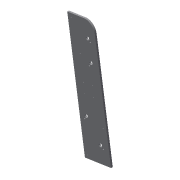
# Autodesk Inventor part: inside wall
Saved by Autodesk Inventor 2020 (Build 240168000, 168)
## iProperties
Created: 2019-10-13
Part Number: inside wall
Material: Generic
Document SubType Name: Modeling
Designer: ball
Density: 1 g/cm^3
Appearance: Default
Author: ball
Autodesk Inventor part; units mm, degrees
ref_plane "YZ Plane" through (0, 0, 0) normal (1, 0, 0) x (0, 1, 0)
ref_plane "XZ Plane" through (0, 0, 0) normal (0, 1, 0) x (-1, 0, 0)
ref_plane "XY Plane" through (0, 0, 0) normal (0, 0, 1) x (1, 0, 0)
ref_plane "Work Plane1" through (-0.0003, 0.0023, 0) normal (0, 0, 1) x (1, 0, 0)
sketch "Sketch1" plane through (-0.0003, 0.0023, 0) normal (0, 0, 1) x (1, 0, 0)
  circle A0 centre (0.0003, -0.0023) radius 6.3373 construction
  circle A1 centre (-49.0975, 326.5271) radius 6.3373 construction
  circle A2 centre (0.0003, -0.0023) radius 6.4135
  circle A3 centre (-49.0975, 326.5271) radius 6.4135
  circle A4 centre (-49.0975, 326.5271) radius 60.325 construction
  circle A5 centre (0.0003, -0.0023) radius 60.325 construction
  circle A6 centre (0.0003, -0.0023) radius 31.75 construction
  line L0 (40.3672, -54.9357) -> (-26.6702, 390.9025)
  circle A7 centre (-49.0975, 326.5271) radius 31.75 construction
  line L1 (-58.7973, -69.8464) -> (40.3672, -54.9357)
  line L2 (-125.8347, 375.9918) -> (-26.6702, 390.9025)
  circle A8 centre (-54.0299, 68.9302) radius 6.3373 construction
  circle A9 centre (-36.6118, 251.3479) radius 6.3373 construction
  circle A10 centre (-54.0299, 68.9302) radius 6.35
  circle A11 centre (-36.6118, 251.3479) radius 6.35
  line L3 (-82.6344, 131.3852) -> (-87.6899, 165.0073) construction
  line L4 (-58.7973, -69.8464) -> (-125.8347, 375.9918)
  point P0 (0.0003, -0.0023)
  dimension "d0" = 12.827
  dimension "d3" = 12.827
  dimension "d11" = 120.65
  dimension "d13" = 120.65
  dimension "d14" = 63.5
  dimension "d16" = 63.5
  dimension "d19" = 12.7
  dimension "d20" = 12.7
  constraints: 10 end point, 8 centre point, 8 coincident, 4 tangent, 3 other
  measures "d0" diameter of A2
  measures "d3" diameter of A3
  measures "d11" diameter of A4
  measures "d13" diameter of A5
  measures "d14" diameter of A6
  measures "d16" diameter of A7
  measures "d19" diameter of A10
  measures "d20" diameter of A11
extrude "Extrusion1" add sketch "Sketch1" along normal blind 6.35
sketch "Sketch2" plane through (-0.0003, 0.0023, 0) normal (0, 0, -1) x (-1, 0, 0)
  circle A0 centre (111.3879, 365.3242) radius 1.778 construction
  circle A1 centre (77.9428, 262.471) radius 1.778 construction
  circle A2 centre (31.0502, 180.1901) radius 1.778 construction
  circle A3 centre (64.857, 175.1068) radius 1.778 construction
  circle A4 centre (25.7636, 145.0307) radius 1.778 construction
  circle A5 centre (59.5704, 139.9475) radius 1.778 construction
  circle A6 centre (48.1268, -55.3992) radius 1.778 construction
  circle A7 centre (111.3879, 365.3242) radius 1.778
  circle A8 centre (77.9428, 262.471) radius 1.778
  circle A9 centre (64.857, 175.1068) radius 1.778
  circle A10 centre (59.5704, 139.9475) radius 1.778
  circle A11 centre (31.0502, 180.1901) radius 1.778
  circle A12 centre (25.7636, 145.0307) radius 1.778
  circle A13 centre (48.1268, -55.3992) radius 1.778
  point P0 (-0.0003, -0.0023)
extrude "Extrusion2" cut sketch "Sketch2" against normal through all
sketch "Sketch3" plane through (-0.0003, 0.0023, 0) normal (0, 0, -1) x (-1, 0, 0)
  circle A0 centre (-7.8664, -5.812) radius 2.8702 construction
  circle A1 centre (58.7683, 60.3758) radius 2.8702 construction
  circle A2 centre (41.3502, 242.7936) radius 2.8702 projected
  circle A3 centre (41.2314, 320.7173) radius 2.8702 construction
  circle A4 centre (39.1236, 318.7692) radius 2.9567
  circle A5 centre (42.9235, 240.393) radius 2.8702
  circle A6 centre (60.507, 58.0922) radius 2.8702
  circle A7 centre (-10.0879, -7.6295) radius 2.8702
  point P0 (-0.0003, -0.0023)
  constraints: 1 centre point, 17 other
extrude "Extrusion3" cut sketch "Sketch3" against normal through all contours A2 A5 | A2 A5 | A4 | A6 | A7 picked at (41.9477, 242.03) picked at (43.9052, 238.7756)
sketch "Sketch4" plane through (-0.0003, 0.0023, 0) normal (0, 0, -1) x (-1, 0, 0)
  arc A0 (58.0673, 386.1815) -> (21.1234, 354.0125) centre (58.7307, 348.1214) ccw construction
  arc A1 (58.0673, 386.1815) -> (21.1234, 354.0125) centre (58.7307, 348.1214) ccw
  line L0 (26.6702, 390.9025) -> (125.8347, 375.9918) projected
  line L1 (58.0673, 386.1815) -> (26.6702, 390.9025)
  line L2 (26.6702, 390.9025) -> (21.1234, 354.0125)
  point P0 (-0.0003, -0.0023)
  constraints: 4 end point, 2 point on circle, 1 centre point, 1 coincident, 1 collinear, 1 perpendicular
extrude "Extrusion4" cut sketch "Sketch4" against normal through all
sketch "Sketch5" plane through (-0.0003, 0.0023, 0) normal (0, 0, -1) x (-1, 0, 0)
  circle A0 centre (-9.1502, 60.0002) radius 2.25 construction
  circle A1 centre (-9.1502, 60.0002) radius 1.8542
  point P0 (-0.0003, -0.0023)
  dimension "d30" = 3.7084
  constraints: 2 centre point, 1 coincident, 2 other
  measures "d30" diameter of A1
extrude "Extrusion5" cut sketch "Sketch5" against normal through all
sketch "Sketch6" plane through (-0.0003, 0.0023, 0) normal (0, 0, -1) x (-1, 0, 0)
  line L0 (-6.9196, 56.5789) -> (-27.6054, 48.4519) construction
  line L1 (-23.0039, 33.2159) -> (-17.622, 69.0087) construction
  line L2 (-40.3672, -54.9357) -> (21.1234, 354.0125) construction
  circle A0 centre (-19.2051, 50.473) radius 1.1906
  point P0 (-0.0003, -0.0023)
  dimension "d33" = 2.3813
  constraints: 4 end point, 2 tangent, 1 centre point, 1 parallel, 3 other
  measures "d33" diameter of A0
extrude "Extrusion6" cut sketch "Sketch6" against normal through all
body "Solid1"
